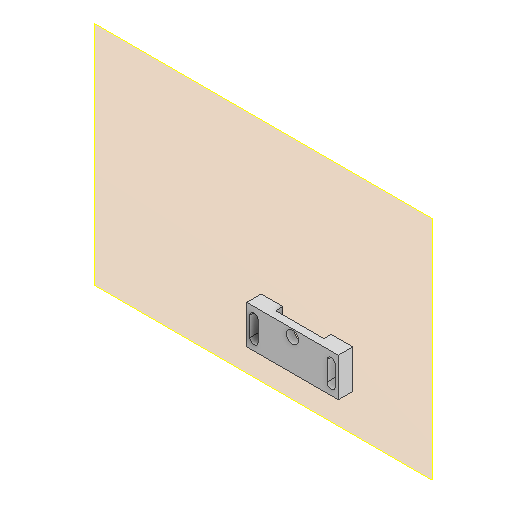
# Autodesk Inventor part: 10_LED_cylnderlensmount
Saved by Autodesk Inventor 2022 (Build 260153000, 153)
## iProperties
Created: 2022-04-18
Part Number: 10_LED_cylnderlensmount
Material: Generic
Document SubType Name: Modeling
Designer: Prakash Lab
Density: 1 g/cm^3
Appearance: Default
Author: Prakash Lab
Autodesk Inventor part; units mm, degrees
ref_plane "YZ Plane" through (0, 0, 0) normal (1, 0, 0) x (0, 1, 0)
ref_plane "XZ Plane" through (0, 0, 0) normal (0, 1, 0) x (-1, 0, 0)
ref_plane "XY Plane" through (0, 0, 0) normal (0, 0, 1) x (1, 0, 0)
ref_plane "Work Plane1" through (0, 0, 0) normal (0, 0, 1) x (1, 0, 0)
sketch "Sketch1" plane through (0, 0, 0) normal (0, 0, 1) x (1, 0, 0)
  circle A0 centre (2.4, -23.5737) radius 1.4 projected
  circle A1 centre (34.4, -23.5737) radius 1.4 projected
  line L0 (2.4, -27.5737) -> (2.4, -19.5737) construction
  line L1 (4.1, -27.5737) -> (4.1, -19.5737)
  line L2 (0.7, -19.5737) -> (0.7, -27.5737)
  arc A2 (0.7, -27.5737) -> (4.1, -27.5737) centre (2.4, -27.5737) ccw
  arc A3 (4.1, -19.5737) -> (0.7, -19.5737) centre (2.4, -19.5737) ccw
  line L3 (34.4, -19.5737) -> (34.4, -27.5737) construction
  line L4 (32.7, -19.5737) -> (32.7, -27.5737)
  line L5 (36.1, -27.5737) -> (36.1, -19.5737)
  arc A4 (36.1, -19.5737) -> (32.7, -19.5737) centre (34.4, -19.5737) ccw
  arc A5 (32.7, -27.5737) -> (36.1, -27.5737) centre (34.4, -27.5737) ccw
  line L6 (-0.6, -31.5737) -> (8.4, -31.5737)
  line L7 (8.4, -31.5737) -> (8.4, -15.5737)
  line L8 (8.4, -15.5737) -> (-0.6, -15.5737)
  line L9 (-0.6, -15.5737) -> (-0.6, -31.5737)
  line L10 (37.4, -15.5737) -> (28.4, -15.5737)
  line L11 (28.4, -15.5737) -> (28.4, -31.5737)
  line L12 (28.4, -31.5737) -> (37.4, -31.5737)
  line L13 (37.4, -31.5737) -> (37.4, -15.5737)
  line L14 (8.4, -7.25) -> (8.4, -25.25)
  line L15 (28.4, -7.25) -> (28.4, -25.25)
  point P0 (0, 0)
  dimension "d0" = 4
  dimension "d1" = 3.4
  dimension "d2" = 3.4
  dimension "d3" = 0
  dimension "d4" = 9
  dimension "d5" = 9
  dimension "d6" = 0
  dimension "d7" = 0
  dimension "d8" = 4
  dimension "d9" = 4
  constraints: 36 end point, 8 point on circle, 8 tangent, 7 parallel, 4 centre point, 3 vertical, 2 horizontal, 2 midpoint, 2 perpendicular, 2 point on line, 4 other
  measures "d0" distance of A0.centre L0.end
  measures "d1" diameter of A3
  measures "d2" diameter of A5
  measures "d3" vertical distance of L0.start L3.end
  measures "d4" distance between parallel lines of L9 L7
  measures "d5" distance between parallel lines of L13 L11
  measures "d6" distance between parallel lines of L6 L12
  measures "d7" distance between parallel lines of L10 L8
  measures "d8" distance from line of L6 L0.start
  measures "d9" distance from line of L8 L0.end
extrude "Extrusion1" add sketch "Sketch1" along normal blind 3 contours L9 L8 L7 L6 | L13 L12 L11 L10
sketch "Sketch2" plane through (0, 0, 3) normal (0, 0, 1) x (1, 0, 0)
  line L0 (8.4, -31.5737) -> (8.4, -15.5737) projected
  line L1 (8.4, -15.5737) -> (-0.6, -15.5737) projected
  line L2 (-0.6, -15.5737) -> (-0.6, -31.5737) projected
  line L3 (-0.6, -31.5737) -> (8.4, -31.5737) projected
  arc A0 (0.7, -27.5737) -> (4.1, -27.5737) centre (2.4, -27.5737) ccw projected
  line L4 (0.7, -27.5737) -> (0.7, -19.5737) projected
  arc A1 (4.1, -19.5737) -> (0.7, -19.5737) centre (2.4, -19.5737) ccw projected
  line L5 (4.1, -19.5737) -> (4.1, -27.5737) projected
  line L6 (37.4, -15.5737) -> (28.4, -15.5737) projected
  line L7 (28.4, -15.5737) -> (28.4, -31.5737) projected
  line L8 (28.4, -31.5737) -> (37.4, -31.5737) projected
  line L9 (37.4, -31.5737) -> (37.4, -15.5737) projected
  arc A2 (36.1, -19.5737) -> (32.7, -19.5737) centre (34.4, -19.5737) ccw projected
  line L10 (36.1, -19.5737) -> (36.1, -27.5737) projected
  arc A3 (32.7, -27.5737) -> (36.1, -27.5737) centre (34.4, -27.5737) ccw projected
  line L11 (32.7, -27.5737) -> (32.7, -19.5737) projected
  line L12 (12.4, 1.5154) -> (12.4, -15.3846)
  line L13 (24.4, 1.5154) -> (24.4, -15.3846)
  circle A4 centre (18.4, -18.5737) radius 2.5
  line L14 (8.4, -15.5737) -> (28.4, -15.5737)
  line L15 (28.4, -31.5737) -> (8.4, -31.5737)
  point P0 (0, 0)
  dimension "d12" = 5
  dimension "d13" = 6
  dimension "d14" = 3
  constraints: 8 end point, 2 vertical, 1 centre point, 1 horizontal, 1 parallel, 4 other
  measures "d12" diameter of A4
  measures "d13" distance from line of A4.centre L12
  measures "d14" distance from line of A4.centre L6
extrude "Extrusion2" add sketch "Sketch2" along normal blind 3
body "Solid1"
